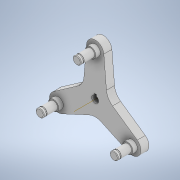
# Autodesk Inventor part: Shaft_interstage
Saved by Autodesk Inventor 2020 (Build 240168000, 168)
## iProperties
Created: 2020-05-11
Part Number: Shaft_interstage
Material: Generic
Document SubType Name: Modeling
Designer: avi41
Density: 1 g/cm^3
Appearance: Default
Author: avi41
Autodesk Inventor part; units mm, degrees
ref_plane "YZ Plane" through (0, 0, 0) normal (1, 0, 0) x (0, 1, 0)
ref_plane "XZ Plane" through (0, 0, 0) normal (0, 1, 0) x (-1, 0, 0)
ref_plane "XY Plane" through (0, 0, 0) normal (0, 0, 1) x (1, 0, 0)
sketch "Sketch1" plane through (0, 0, 0) normal (0, 1, 0) x (-1, 0, 0)
  line L0 (0, -16.1) -> (0, 16.1) construction
  line L1 (-54, 0) -> (9, 0) construction
  line L2 (-3, 11.5) -> (-45, 11.5)
  line L3 (-45, 11.5) -> (-45, -11.5)
  line L4 (-45, -11.5) -> (-3, -11.5)
  line L5 (-3, -11.5) -> (-3, 11.5)
  point P0 (0, 0)
  dimension "d1" = 23
  dimension "d4" = 45
  dimension "d36" = 3
  constraints: 8 end point, 3 perpendicular, 1 horizontal, 1 point on line, 1 other
  measures "d1" distance of L2.end L3.end
  measures "d4" distance between parallel lines of L0 L3
  measures "d36" distance between parallel lines of L0 L5
revolve "Revolution1" add sketch "Sketch1" angle 360 about axis through (0, 0, 0) along (0, 0, 1)
sketch "Sketch2" plane through (0, 0, -11.5) normal (0, 0, -1) x (-1, 0, 0)
  line L0 (0, -63.2055) -> (0, 64.2333) construction
  line L1 (-63, 0) -> (63, 0) construction
  arc A0 (7.4715, 37.7287) -> (0, 44.575) centre (0, 37.075) ccw
  line L2 (0, 0) -> (38.9711, -22.5) construction
  circle A1 centre (0, 0) radius 45 projected
  line L3 (0, 0) -> (-38.9711, -22.5) construction
  line L4 (0, 0) -> (38.9711, 22.5)
  arc A2 (9.7463, 11.727) -> (11.3734, 6.5665) centre (22.1987, 12.8165) ccw
  line L5 (7.4715, 37.7287) -> (9.7463, 11.727)
  arc A3 (0, 44.575) -> (-7.4715, 37.7287) centre (0, 37.075) ccw
  arc A4 (-11.3734, 6.5665) -> (-9.7463, 11.727) centre (-22.1987, 12.8165) ccw
  line L6 (-7.4715, 37.7287) -> (-9.7463, 11.727)
  line L7 (0, 0) -> (-2.1651, 1.25)
  line L8 (-11.3734, 6.5665) -> (-38.9711, 22.5)
  point P0 (-38.9711, 22.5)
  point P1 (0, 45)
  point P2 (0, 45)
  dimension "d6" = 15
  dimension "d7" = 120
  dimension "d8" = 120
  dimension "d9" = 60
  dimension "d10" = 60
  dimension "d11" = 37.075
  dimension "d12" = 25
  dimension "d13" = 5
  constraints: 14 end point, 11 point on circle, 5 symmetric about line, 4 centre point, 4 point on line, 2 tangent, 1 coincident, 2 other
  measures "d6" diameter of A0
  measures "d7" angle of L0 L3
  measures "d8" angle of L0 L2
  measures "d9" angle of L4 L0
  measures "d10" angle of L2 L4
  measures "d11" distance from line of L1 A0.centre
  measures "d12" diameter of A2
  measures "d13" angle of L5 L0
extrude "Extrusion1" cut sketch "Sketch2" against normal through all contours A0 A3 L6 A4 L8 A1 L4 A2 L5 picked at (-14.556, 28.6205)
sketch "Sketch4" plane through (0, 0, 11.5) normal (0, 0, 1) x (1, 0, 0)
  line L0 (38.9711, 22.5) -> (11.3734, 6.5665) projected
  arc A0 (9.7463, 11.727) -> (11.3734, 6.5665) centre (22.1987, 12.8165) ccw projected
  line L1 (9.7463, 11.727) -> (7.4715, 37.7287) projected
  arc A1 (7.4715, 37.7287) -> (-7.4715, 37.7287) centre (0, 37.075) ccw projected
  line L2 (-7.4715, 37.7287) -> (-9.7463, 11.727) projected
  arc A2 (-11.3734, 6.5665) -> (-9.7463, 11.727) centre (-22.1987, 12.8165) ccw projected
  line L3 (-11.3734, 6.5665) -> (-38.9711, 22.5) projected
  arc A3 (-38.9711, 22.5) -> (38.9711, 22.5) centre (0, 0) ccw projected
  circle A4 centre (0, 37.075) radius 4.5
  line L4 (-38.9711, 22.5) -> (0, 0)
  line L5 (0, 0) -> (38.9711, 22.5)
  circle A5 centre (0, 37.075) radius 3.5
  point P0 (-11.3734, 6.5665)
  dimension "d20" = 9
  dimension "d23" = 7
  constraints: 4 end point, 2 centre point, 2 coincident, 1 point on circle
  measures "d20" diameter of A4
  measures "d23" diameter of A5
extrude "Extrusion2" cut sketch "Sketch4" against normal blind 16 contours L5 L4 A2 L2 A1 L1 A0
extrude "Extrusion4" cut sketch "Sketch4" against normal blind 12 contours A4
sketch "Sketch6" plane through (0, 0, 0) normal (1, 0, 0) x (0, 1, 0)
  line L0 (40.575, -0.5) -> (33.575, -0.5) projected
  line L1 (40.575, 11.5) -> (33.575, 11.5) projected
  line L2 (33.575, -0.5) -> (33.575, 11.5) projected
  line L3 (40.575, -0.5) -> (40.575, 11.5) projected
  line L4 (40.575, 9.4) -> (40.375, 9.4)
  line L5 (40.375, 9.4) -> (40.375, 8.5)
  line L6 (40.375, 8.5) -> (40.575, 8.5)
  line L7 (40.575, 8.5) -> (40.575, 9.4)
  line L8 (37.075, 16.1) -> (37.075, -16.1) projected
  point P0 (0, 0)
  dimension "d29" = 9
  dimension "d34" = 6.8
  dimension "d35" = 0.9
  constraints: 8 end point, 2 parallel, 1 horizontal, 1 perpendicular, 1 point on line
  measures "d29" distance between parallel lines of L0 L6
  measures "d34" distance between parallel lines of L2 L5
  measures "d35" distance between parallel lines of L6 L4
revolve "Revolution2" cut sketch "Sketch6" angle 360 about axis through (0, 37.075, 11.5) along (0, 0, -1) contours L6 L5 L4 L3
chamfer "Chamfer1" distance 0.5 angle 45 1 edges at (-3.5, 37.075, 11.5)
pattern_circular "Circular Pattern1" count 3 over 360 about axis through (0, 0, -10) along (0, 0, 1) of "Extrusion1", "Extrusion2", "Extrusion4", "Revolution2", "Chamfer1"
sketch "Sketch7" plane through (0, 0, -4.5) normal (0, 0, 1) x (1, 0, 0)
  circle A0 centre (0, 0) radius 3 construction
  line L0 (-1, 4.2) -> (1, 4.2)
  line L1 (1, 4.2) -> (1, 2)
  line L2 (1, 2) -> (-1, 2)
  line L3 (-1, 2) -> (-1, 4.2)
  line L4 (0, 58.6975) -> (0, -40.16) construction
  line L5 (-55.451, 0) -> (55.451, 0) construction
  dimension "d37" = 2
  dimension "d38" = 2.2
  dimension "d39" = 2
  constraints: 8 end point, 2 parallel, 1 horizontal, 1 perpendicular, 1 other
  measures "d37" distance between parallel lines of L5 L2
  measures "d38" distance between parallel lines of L2 L0
  measures "d39" distance of L0.start L0.end
extrude "Extrusion5" cut sketch "Sketch7" against normal through all
equation "\"d9\" = d10"
body "Solid1"
